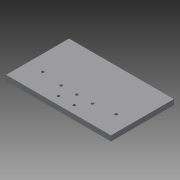
# Autodesk Inventor part: tractor
Saved by Autodesk Inventor 2013 (Build 170138000, 138)
## iProperties
Created: 2012-11-28
Part Number: tractor
Material: Generic
Document SubType Name: Modeling
Designer: Istvan
Density: 1 g/cm^3
Mass: 475.52 g
Surface Area: 904.604 cm^2
Volume: 475.52 cm^3
Author: Istvan
Autodesk Inventor part; units mm, degrees
ref_plane "YZ Plane" through (0, 0, 0) normal (1, 0, 0) x (0, 1, 0)
ref_plane "XZ Plane" through (0, 0, 0) normal (0, 1, 0) x (-1, 0, 0)
ref_plane "XY Plane" through (0, 0, 0) normal (0, 0, 1) x (1, 0, 0)
sketch "Sketch1" plane through (0, 0, 0) normal (0, 1, 0) x (-1, 0, 0)
  line L0 (0, 0) -> (254, 0)
  line L1 (254, 0) -> (254, 152.4)
  line L2 (254, 152.4) -> (0, 152.4)
  line L3 (0, 152.4) -> (0, 0)
  dimension "d0" = 254
  dimension "d1" = 152.4
  constraints: 8 end point, 2 parallel, 1 horizontal, 1 perpendicular
  measures "d0" distance of L2.end L1.end
  measures "d1" distance of L1.end L0.end
extrude "Extrusion1" add sketch "Sketch1" against normal blind 12.7
sketch "Sketch5" plane through (0, -12.7, 0) normal (0, -1, 0) x (1, 0, 0)
  line L0 (0, 0) -> (0, 152.4) projected
  line L1 (0, 152.4) -> (-254, 152.4) projected
  line L2 (-254, 152.4) -> (-254, 0) projected
  point P0 (-38.1, 101.6)
  point P1 (-215.9, 101.6)
  dimension "d20" = 50.8
  dimension "d21" = 38.1
  dimension "d22" = 38.1
  constraints: 1 horizontal alignment
  measures "d20" distance from line of L1 point (-215.9, 101.6)
  measures "d21" distance from line of L2 point (-215.9, 101.6)
  measures "d22" distance from line of L0 point (-38.1, 101.6)
hole "Hole1" at (-38.1, -12.7, 101.6) at (-215.9, -12.7, 101.6) direction (0, 1, 0) diameter 6.35 end through all
sketch "Sketch10" plane through (0, 0, 0) normal (0, 1, 0) x (1, 0, 0)
  line L0 (-254, 0) -> (-254, -152.4) projected
  line L1 (-254, -152.4) -> (0, -152.4) projected
  line L2 (0, -152.4) -> (0, 0) projected
  point P0 (-88.9, -107.95)
  point P1 (-127, -107.95)
  point P2 (-165.1, -107.95)
  point P3 (-146.05, -133.35)
  point P4 (-107.95, -133.35)
  dimension "d67" = 38.1
  dimension "d69" = 38.1
  dimension "d70" = 19.05
  dimension "d71" = 19.05
  dimension "d72" = 127
  dimension "d73" = 127
  dimension "d74" = 19.05
  dimension "d75" = 25.4
  constraints: 3 horizontal alignment
  measures "d67" distance of point (-88.9, -107.95) point (-127, -107.95)
  measures "d69" distance of point (-165.1, -107.95) point (-127, -107.95)
  measures "d70" horizontal distance of point (-107.95, -133.35) point (-127, -107.95)
  measures "d71" horizontal distance of point (-146.05, -133.35) point (-127, -107.95)
  measures "d72" distance from line of L0 point (-127, -107.95)
  measures "d73" distance from line of L2 point (-127, -107.95)
  measures "d74" distance from line of L1 point (-146.05, -133.35)
  measures "d75" vertical distance of point (-165.1, -107.95) point (-146.05, -133.35)
hole "Hole5" at (-88.9, 0, 107.95) at (-127, 0, 107.95) at (-165.1, 0, 107.95) at (-146.05, 0, 133.35) at (-107.95, 0, 133.35) direction (0, -1, 0) diameter 6.35 end through all
equation "\"d22\" = d21"
equation "\"d72\" = d73"
body "Solid1"
